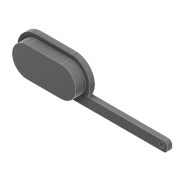
# Autodesk Inventor part: tappino tpu
Saved by Autodesk Inventor 2022 (Build 260153000, 153)
## iProperties
Created: 2025-08-17
Part Number: tappino tpu
Material: Thermoplastic Resin
Document SubType Name: Modeling
Designer: sacchie
Density: 1.28 g/cm^3
Appearance: Smooth - Black
Author: sacchie
Autodesk Inventor part; units mm, degrees
ref_plane "YZ Plane" through (0, 0, 0) normal (1, 0, 0) x (0, 1, 0)
ref_plane "XZ Plane" through (0, 0, 0) normal (0, 1, 0) x (-1, 0, 0)
ref_plane "XY Plane" through (0, 0, 0) normal (0, 0, 1) x (1, 0, 0)
sketch "Sketch1" plane through (0, 0, 0) normal (0, 0, 1) x (1, 0, 0)
  line L0 (0, 0) -> (-7, 0) construction
  line L1 (0, 4) -> (-7, 4)
  line L2 (-7, -4) -> (0, -4)
  arc A0 (0, -4) -> (0, 4) centre (0, 0) ccw
  arc A1 (-7, 4) -> (-7, -4) centre (-7, 0) ccw
  line L3 (-7, 3.1) -> (0, 3.1)
  arc A2 (0, -3.1) -> (0, 3.1) centre (0, 0) ccw
  line L4 (0, -3.1) -> (-7, -3.1)
  arc A3 (-7, 3.1) -> (-7, -3.1) centre (-7, 0) ccw
  line L5 (0, -4) -> (19.2, -4)
  line L6 (20, -3.2) -> (20, -2.8)
  line L7 (19.2, -2) -> (3.4641, -2)
  circle A4 centre (18.8, -3) radius 0.5
  arc A5 (20, -2.8) -> (19.2, -2) centre (19.2, -2.8) ccw
  arc A6 (19.2, -4) -> (20, -3.2) centre (19.2, -3.2) ccw
  point P0 (-3.5, 0)
  point P1 (20, -4)
  point P2 (20, -2)
  dimension "d0" = 7
  dimension "d1" = 8
  dimension "d5" = 3.1
  dimension "d6" = 2
  dimension "d7" = 1
  dimension "d8" = 20
  dimension "d9" = 1.2
  dimension "d10" = 0.8
  constraints: 18 end point, 13 point on circle, 8 tangent, 7 centre point, 4 point on line, 2 horizontal, 2 parallel, 2 perpendicular, 1 equal radius, 1 midpoint, 3 other
  measures "d0" distance of L0.start L0.end
  measures "d1" diameter of A1
  measures "d5" radius of A2
  measures "d6" distance of point (20, -4) point (20, -2)
  measures "d7" diameter of A4
  measures "d8" distance from line of L0.start L6
  measures "d9" distance from line of L6 A4.centre
  measures "d10" radius of A5
extrude "Extrusion1" add sketch "Sketch1" along normal blind 1 contours A0 L2 A1 L1 | L7 A5 L6 A6 L5 A0 | L3 A2 L4 A3
extrude "Extrusion2" add sketch "Sketch1" along normal blind 2 from surface at 1 contours L3 A2 L4 A3
body "Solid1"
